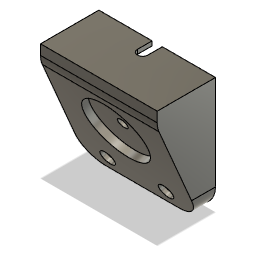
simple knob box base (Autodesk Fusion 360 design; units mm, degrees)
Autodesk Fusion 360 part; units mm, degrees
note: some values were not read from the file. Set by a fixed rule: which face or edge a step refers to.
sketch "Sketch1" plane through (0, 0, 0) normal (0, 0, 1) x (1, 0, 0)
  line L0 (-40, 40) -> (40, 40)
  line L1 (40, 40) -> (40, -40)
  line L2 (40, -40) -> (-40, -40)
  line L3 (-40, -40) -> (-40, 40)
  point P0 (0, 40)
  point P1 (-40, 0)
  dimension "d1" = 80
  dimension "d2" = 80
  constraint horizontal L0
  constraint vertical L1
  constraint horizontal L2
  constraint vertical L3
  constraint midpoint L0 P0
  constraint vertical origin P0
  constraint midpoint L3 P1
  constraint horizontal origin P1
  measures "d1" distance of L0.start L0.end
  measures "d2" distance of L0.start L2.end
extrude "Extrude1" add sketch "Sketch1" along normal blind 40
sketch "Sketch2" plane through (40, 0, 0) normal (1, 0, 0) x (0, 0, -1)
  line L0 (0, -40) -> (0, 40)
  line L1 (0, 40) -> (-40, 40)
  line L2 (-40, 40) -> (-40, -40)
  line L3 (-40, -40) -> (0, -40)
  line L4 (-40, 30) -> (-10, -40)
  dimension "d5" = 30
  dimension "d31" = 10
  constraint coincident L2 L4.start
  constraint coincident L3 L4.end
  measures "d5" distance of L2.end L4.end
  measures "d31" distance of L1.end L4.start
extrude "Extrude2" cut sketch "Sketch2" against normal up to surface (80 mm away) contours L2 L3 L4
sketch "Sketch3" plane through (0, -9.8276, 22.931) normal (0, -0.393919, 0.919145) x (1, 0, 0)
  line L0 (-40, 43.3311) -> (-40, -32.8266)
  line L1 (-40, -32.8266) -> (40, -32.8266)
  line L2 (40, -32.8266) -> (40, 43.3311)
  line L3 (40, 43.3311) -> (-40, 43.3311)
  circle A0 centre (0, 13.3311) radius 20
  circle A1 centre (0, 13.3311) radius 22
  dimension "d9" = 40
  dimension "d10" = 30
  dimension "d11" = 2
  constraint vertical origin A0.centre
  measures "d9" diameter of A0
  measures "d10" distance of L3 A0.centre
extrude "Extrude3" cut sketch "Sketch3" against normal blind 5 contours A0 | A1
sketch "Sketch4" plane through (0, -7.858, 18.3353) normal (0, -0.393919, 0.919145) x (1, 0, 0)
  circle A0 centre (0, 13.3311) radius 22
  circle A1 centre (0, 13.3311) radius 3.5
  dimension "d14" = 7
  constraint concentric A0 A1
  measures "d14" diameter of A1
shell "Shell1" thickness 3 removed faces 1 at (-13.3333, 13.3333, 0)
extrude "Extrude4" cut sketch "Sketch4" against normal up to surface (3 mm away) contours A1
sketch "Sketch5" plane through (0, -9.8276, 22.931) normal (0, -0.393919, 0.919145) x (1, 0, 0)
  circle A0 centre (0, 13.3311) radius 22
  line L0 (-40, 43.3311) -> (-40, -32.8266)
  line L1 (-40, -32.8266) -> (40, -32.8266)
  line L2 (40, -32.8266) -> (40, 43.3311)
  line L3 (40, 43.3311) -> (-40, 43.3311)
  circle A1 centre (-20, -22.8266) radius 5
  circle A2 centre (20, -22.8266) radius 5
  line L4 (-20, -22.8266) -> (20, -22.8266) construction
  point P0 (0, -22.8266)
  dimension "d18" = 10
  dimension "d19" = 10
  dimension "d20" = 10
  dimension "d21" = 40
  constraint coincident A1.centre L4.start
  constraint coincident A2.centre L4.end
  constraint horizontal L4
  constraint midpoint L4 P0
  constraint vertical A0.centre P0
  measures "d18" distance of L1 L4
  measures "d19" diameter of A1
  measures "d20" diameter of A2
  measures "d21" distance of A1.centre A2.centre
extrude "Extrude5" cut sketch "Sketch5" against normal up to surface (3 mm away) contours A1 | A2
sketch "Sketch6" plane through (0, 40, 0) normal (0, 1, 0) x (-1, 0, 0)
  line L0 (-40, 0) -> (40, 0)
  line L1 (40, 0) -> (40, 40)
  line L2 (40, 40) -> (-40, 40)
  line L3 (-40, 40) -> (-40, 0)
  circle A0 centre (0, 10) radius 3.5
  line L4 (-3.5, 10) -> (-3.5, 0)
  line L5 (3.5, 10) -> (3.5, 0)
  dimension "d24" = 7
  dimension "d25" = 10
  constraint coincident A0 L4.start
  constraint coincident L0 L4.end
  constraint coincident A0 L5.start
  constraint coincident L0 L5.end
  constraint tangent A0 L5
  constraint tangent A0 L4
  constraint vertical L4
  constraint vertical L5
  constraint vertical origin A0.centre
  measures "d24" diameter of A0
  measures "d25" distance of L4.start L4.end
extrude "Extrude6" cut sketch "Sketch6" against normal up to surface (3 mm away) contours L0 A0 L4 L5 | A0
fillet "Fillet1" radius 15 4 edges at (-40, -40, 5) (40, -40, 5) (37, -37, 4.0109) (-37, -37, 4.0109)
fillet "Fillet2" radius 15 2 edges at (0, 30, 40) (0, 37, 37)
sketch "Sketch7" plane through (0, -6.6762, 15.5779) normal (0, 0.393919, -0.919145) x (-1, 0, 0)
  circle A0 centre (0, 13.3311) radius 3.5
  circle A1 centre (0, 13.3311) radius 25
extrude "Extrude7" add sketch "Sketch7" along normal blind 7
equation "d20 = d19"
